2.5mm top thick (Autodesk Fusion 360 design; units mm, degrees)
Autodesk Fusion 360 part; units mm, degrees
note: some values were not read from the file. Chosen so that the rebuilt part matches the saved one: which bodies a step acts on. Set by a fixed rule: which sketch regions a step uses.
sketch "Sketch1" plane through (0, 0, 0) normal (0, 0, 1) x (1, 0, 0)
  line L0 (-31.9745, -0.1006) -> (0, 0) construction
  line L1 (0, 0) -> (-0.051, 16.2012) construction
  line L2 (-0.051, 16.2012) -> (-32.0255, 16.1006) construction
  line L3 (-32.0255, 16.1006) -> (-31.9745, -0.1006) construction
  dimension "d1" = 3
  text T0 "2.5 mm top thick" font "Arial" height 3 align right bottom in box 31.9747 x 16.2013 at (-31.9745, -0.1006) x (0.999995, 0.003146) y (-0.003146, 0.999995) spacing 1
  constraint coincident L0.end
extrude "Extrude1" add sketch "Sketch1" along normal blind 1 text T0 makes body 1 at (-23.3424, 1.0268, 0) makes body 2 at (-26.1166, 2.7596, 0) makes body 3 at (-29.7703, 0.0244, 0) makes body 4 at (-7.1634, 0.9775, 0.3333) makes body 5 at (-8.0162, 1.0212, 0) makes body 6 at (-1.804, 0.9943, 0.3333) makes body 7 at (-14.1543, 1.1923, 0) makes body 8 at (-19.8512, 1.0378, 0) makes body 9 at (-28.0174, 0.0517, 0.3333) makes body 10 at (-15.0066, 0.9992, 0) makes body 11 at (-11.8204, 0.132, 0.3333) makes body 12 at (-4.8359, 2.7024, 0.3333) makes body 13 at (-3.7205, 0.4174, 0) makes body 14 at (-4.8297, 0.7092, 0.3333)
sketch "Sketch2" plane through (0, 0, 0) normal (0, 0, 1) x (1, 0, 0)
  line L0 (-30, 4.2795) -> (0.5307, 4.2795)
  line L1 (0.5307, 4.2795) -> (0.5307, -1.4537)
  line L2 (0.5307, -1.4537) -> (-30, -1.4537)
  line L3 (-30, -1.4537) -> (-30, 4.2795)
  circle A0 centre (0.5307, 1.4129) radius 2.8666
  circle A1 centre (-30, 1.4129) radius 2.8666
  constraint horizontal L0
  constraint vertical L1
  constraint horizontal L2
  constraint vertical L3
  constraint coincident L1.end A0
  constraint tangent L2 A0
  constraint coincident L0.end A0
  constraint coincident L2.end A1
  constraint tangent L2 A1
  constraint coincident L0.start A1
extrude "Extrude2" add sketch "Sketch2" against normal blind 1 bodies 1 2 3
